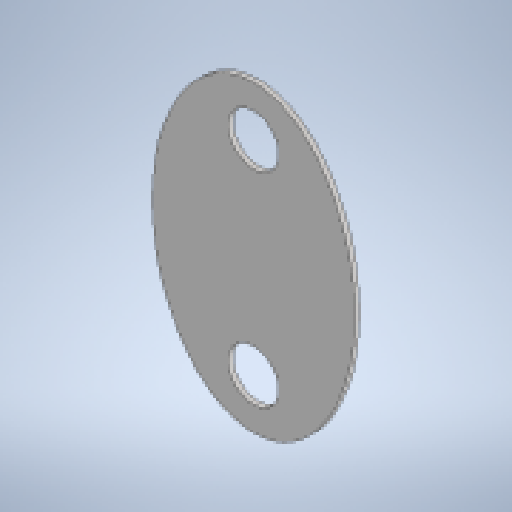
# Autodesk Inventor part: нижний эллипс тела
Saved by Autodesk Inventor 2023.1 (Build 271208000, 208)
## iProperties
Created: 2024-11-21
Part Number: нижний эллипс тела
Material: Типовые
Document SubType Name: Modeling
Designer: DELL
Density: 1 g/cm^3
Appearance: По умолчанию
Author: DELL
Autodesk Inventor part; units mm, degrees
ref_plane "YZ Plane" through (0, 0, 0) normal (1, 0, 0) x (0, 1, 0)
ref_plane "XZ Plane" through (0, 0, 0) normal (0, 1, 0) x (-1, 0, 0)
ref_plane "XY Plane" through (0, 0, 0) normal (0, 0, 1) x (1, 0, 0)
sketch "Эскиз1" plane through (0, 0, 0) normal (0, 0, 1) x (1, 0, 0)
  line L0 (2.6725, 99.2298) -> (22.6725, -99.2298) construction
  ellipse E0 centre (12.6725, 0) end of major axis (12.6725, -120) minor radius 80
  circle A0 centre (0, 225.3213) radius 4 construction
  circle A1 centre (0, -225.3213) radius 4 construction
  arc A2 (-125.6303, -24.4298) -> (-125.6303, -42.4298) centre (-125.6303, -33.4298) ccw construction
  line L1 (-125.6303, -24.4298) -> (-77.5364, -24.4298) construction
  arc A3 (-77.5364, -42.4298) -> (-77.5364, -24.4298) centre (-77.5364, -33.4298) ccw construction
  line L2 (-77.5364, -42.4298) -> (-125.6303, -42.4298) construction
  line L3 (-25, -17) -> (-32, -17) construction
  line L4 (-32, -17) -> (-32, -7) construction
  line L5 (-32, -7) -> (-25, -7) construction
  line L6 (-25, -7) -> (-25, -17) construction
  line L7 (-125.6303, 42.4298) -> (-77.5364, 42.4298) construction
  arc A4 (-77.5364, 24.4298) -> (-77.5364, 42.4298) centre (-77.5364, 33.4298) ccw construction
  line L8 (-77.5364, 24.4298) -> (-125.6303, 24.4298) construction
  arc A5 (-125.6303, 42.4298) -> (-125.6303, 24.4298) centre (-125.6303, 33.4298) ccw construction
  line L9 (-125, 7) -> (-132, 7) construction
  line L10 (-132, 7) -> (-132, 17) construction
  line L11 (-132, 17) -> (-125, 17) construction
  line L12 (-125, 17) -> (-125, 7) construction
  circle A6 centre (159.3262, -159.3262) radius 4 construction
  circle A7 centre (-159.3262, -159.3262) radius 4 construction
  line L13 (22.6725, -100.7298) -> (2.6725, -100.7298) construction
  line L14 (2.6725, -100.7298) -> (2.6725, -60.7298) construction
  line L15 (2.6725, -60.7298) -> (22.6725, -60.7298) construction
  line L16 (22.6725, -60.7298) -> (22.6725, -100.7298) construction
  circle A8 centre (-159.3262, 159.3262) radius 4 construction
  circle A9 centre (225.3213, 0) radius 4 construction
  line L17 (-32, 17) -> (-25, 17) construction
  line L18 (-25, 17) -> (-25, 7) construction
  line L19 (-25, 7) -> (-32, 7) construction
  line L20 (-32, 7) -> (-32, 17) construction
  line L21 (-75, -17) -> (-82, -17) construction
  line L22 (-82, -17) -> (-82, -7) construction
  line L23 (-82, -7) -> (-75, -7) construction
  line L24 (-75, -7) -> (-75, -17) construction
  line L25 (-125, -17) -> (-132, -17) construction
  line L26 (-132, -17) -> (-132, -7) construction
  line L27 (-132, -7) -> (-125, -7) construction
  line L28 (-125, -7) -> (-125, -17) construction
  line L29 (-75, 7) -> (-82, 7) construction
  line L30 (-82, 7) -> (-82, 17) construction
  line L31 (-82, 17) -> (-75, 17) construction
  line L32 (-75, 17) -> (-75, 7) construction
  circle A10 centre (159.3262, 159.3262) radius 4 construction
  circle A11 centre (-225.3213, 0) radius 4 construction
  line L33 (22.6725, 60.7298) -> (2.6725, 60.7298) construction
  line L34 (2.6725, 60.7298) -> (2.6725, 100.7298) construction
  line L35 (2.6725, 100.7298) -> (22.6725, 100.7298) construction
  line L36 (22.6725, 100.7298) -> (22.6725, 60.7298) construction
  circle A12 centre (-104.2556, 141.9298) radius 1.5 construction
  line L37 (-71.1919, 138.9298) -> (-71.1919, 144.9298) construction
  line L38 (-71.1919, 144.9298) -> (-57.9061, 144.9298) construction
  line L39 (-57.9061, 144.9298) -> (-57.9061, 138.9298) construction
  line L40 (-57.9061, 138.9298) -> (-71.1919, 138.9298) construction
  line L41 (-97.7633, 55.9298) -> (-97.7633, 61.9298) construction
  line L42 (-97.7633, 61.9298) -> (-84.4776, 61.9298) construction
  line L43 (-84.4776, 61.9298) -> (-84.4776, 55.9298) construction
  line L44 (-84.4776, 55.9298) -> (-97.7633, 55.9298) construction
  circle A13 centre (-77.5336, 58.9298) radius 1.5 construction
  line L45 (-101.4061, 113.2631) -> (-101.4061, 87.5965) construction
  line L46 (-101.4061, 87.5965) -> (-107.4061, 87.5965) construction
  line L47 (-107.4061, 87.5965) -> (-107.4061, 113.2631) construction
  line L48 (-107.4061, 113.2631) -> (-101.4061, 113.2631) construction
  line L49 (83.8167, 100.7298) -> (83.8167, 106.7298) construction
  line L50 (83.8167, 106.7298) -> (96.6738, 106.7298) construction
  line L51 (96.6738, 106.7298) -> (96.6738, 100.7298) construction
  line L52 (96.6738, 100.7298) -> (83.8167, 100.7298) construction
  line L53 (109.531, 100.7298) -> (109.531, 106.7298) construction
  line L54 (109.531, 106.7298) -> (122.3881, 106.7298) construction
  line L55 (122.3881, 106.7298) -> (122.3881, 100.7298) construction
  line L56 (122.3881, 100.7298) -> (109.531, 100.7298) construction
  circle A14 centre (77.3881, 103.7298) radius 1.5 construction
  circle A15 centre (129.1261, 141.9298) radius 1.5 construction
  line L57 (-84.4776, -138.9298) -> (-84.4776, -144.9298) construction
  line L58 (-84.4776, -144.9298) -> (-97.7633, -144.9298) construction
  line L59 (-97.7633, -144.9298) -> (-97.7633, -138.9298) construction
  line L60 (-97.7633, -138.9298) -> (-84.4776, -138.9298) construction
  line L61 (-71.1919, -55.9298) -> (-57.9061, -55.9298) construction
  line L62 (-57.9061, -55.9298) -> (-57.9061, -61.9298) construction
  line L63 (-57.9061, -61.9298) -> (-71.1919, -61.9298) construction
  line L64 (-71.1919, -61.9298) -> (-71.1919, -55.9298) construction
  circle A16 centre (-77.5336, -141.9298) radius 1.5 construction
  line L65 (135.2452, -100.7298) -> (148.1024, -100.7298) construction
  line L66 (148.1024, -100.7298) -> (148.1024, -106.7298) construction
  line L67 (148.1024, -106.7298) -> (135.2452, -106.7298) construction
  line L68 (135.2452, -106.7298) -> (135.2452, -100.7298) construction
  line L69 (70.9595, -106.7298) -> (58.1024, -106.7298) construction
  line L70 (58.1024, -106.7298) -> (58.1024, -100.7298) construction
  line L71 (58.1024, -100.7298) -> (70.9595, -100.7298) construction
  line L72 (70.9595, -100.7298) -> (70.9595, -106.7298) construction
  circle A17 centre (77.3881, -141.9298) radius 1.5 construction
  line L73 (122.3881, -106.7298) -> (109.531, -106.7298) construction
  line L74 (109.531, -106.7298) -> (109.531, -100.7298) construction
  line L75 (109.531, -100.7298) -> (122.3881, -100.7298) construction
  line L76 (122.3881, -100.7298) -> (122.3881, -106.7298) construction
  line L77 (96.6738, -100.7298) -> (96.6738, -106.7298) construction
  line L78 (96.6738, -106.7298) -> (83.8167, -106.7298) construction
  line L79 (83.8167, -106.7298) -> (83.8167, -100.7298) construction
  line L80 (83.8167, -100.7298) -> (96.6738, -100.7298) construction
  circle A18 centre (103.2571, -141.9298) radius 1.5 construction
  line L81 (135.2452, -144.9298) -> (135.2452, -138.9298) construction
  line L82 (135.2452, -138.9298) -> (148.1024, -138.9298) construction
  line L83 (148.1024, -138.9298) -> (148.1024, -144.9298) construction
  line L84 (148.1024, -144.9298) -> (135.2452, -144.9298) construction
  circle A19 centre (-77.5336, -58.9298) radius 1.5 construction
  circle A20 centre (-104.2556, -141.9298) radius 1.5 construction
  line L85 (-107.4061, -113.2631) -> (-107.4061, -87.5965) construction
  line L86 (-107.4061, -87.5965) -> (-101.4061, -87.5965) construction
  line L87 (-101.4061, -87.5965) -> (-101.4061, -113.2631) construction
  line L88 (-101.4061, -113.2631) -> (-107.4061, -113.2631) construction
  line L89 (-111.049, -138.9298) -> (-111.049, -144.9298) construction
  line L90 (-111.049, -144.9298) -> (-124.3347, -144.9298) construction
  line L91 (-124.3347, -144.9298) -> (-124.3347, -138.9298) construction
  line L92 (-124.3347, -138.9298) -> (-111.049, -138.9298) construction
  circle A21 centre (129.1261, 103.7298) radius 1.5 construction
  circle A22 centre (77.3881, 141.9298) radius 1.5 construction
  line L93 (96.6738, 138.9298) -> (83.8167, 138.9298) construction
  line L94 (83.8167, 138.9298) -> (83.8167, 144.9298) construction
  line L95 (83.8167, 144.9298) -> (96.6738, 144.9298) construction
  line L96 (96.6738, 144.9298) -> (96.6738, 138.9298) construction
  line L97 (135.2452, 100.7298) -> (135.2452, 106.7298) construction
  line L98 (135.2452, 106.7298) -> (148.1024, 106.7298) construction
  line L99 (148.1024, 106.7298) -> (148.1024, 100.7298) construction
  line L100 (148.1024, 100.7298) -> (135.2452, 100.7298) construction
  line L101 (-150.9061, 55.9298) -> (-150.9061, 61.9298) construction
  line L102 (-150.9061, 61.9298) -> (-137.6204, 61.9298) construction
  line L103 (-137.6204, 61.9298) -> (-137.6204, 55.9298) construction
  line L104 (-137.6204, 55.9298) -> (-150.9061, 55.9298) construction
  circle A23 centre (-104.2556, 58.9298) radius 1.5 construction
  circle A24 centre (-130.9776, 141.9298) radius 1.5 construction
  circle A25 centre (-77.5336, 141.9298) radius 1.5 construction
  line L105 (-124.3347, 55.9298) -> (-124.3347, 61.9298) construction
  line L106 (-124.3347, 61.9298) -> (-111.049, 61.9298) construction
  line L107 (-111.049, 61.9298) -> (-111.049, 55.9298) construction
  line L108 (-111.049, 55.9298) -> (-124.3347, 55.9298) construction
  line L109 (-124.3347, 138.9298) -> (-124.3347, 144.9298) construction
  line L110 (-124.3347, 144.9298) -> (-111.049, 144.9298) construction
  line L111 (-111.049, 144.9298) -> (-111.049, 138.9298) construction
  line L112 (-111.049, 138.9298) -> (-124.3347, 138.9298) construction
  line L113 (-97.7633, 144.9298) -> (-84.4776, 144.9298) construction
  line L114 (-84.4776, 144.9298) -> (-84.4776, 138.9298) construction
  line L115 (-84.4776, 138.9298) -> (-97.7633, 138.9298) construction
  line L116 (-97.7633, 138.9298) -> (-97.7633, 144.9298) construction
  line L117 (135.2452, 144.9298) -> (148.1024, 144.9298) construction
  line L118 (148.1024, 144.9298) -> (148.1024, 138.9298) construction
  line L119 (148.1024, 138.9298) -> (135.2452, 138.9298) construction
  line L120 (135.2452, 138.9298) -> (135.2452, 144.9298) construction
  line L121 (70.9595, 144.9298) -> (70.9595, 138.9298) construction
  line L122 (70.9595, 138.9298) -> (58.1024, 138.9298) construction
  line L123 (58.1024, 138.9298) -> (58.1024, 144.9298) construction
  line L124 (58.1024, 144.9298) -> (70.9595, 144.9298) construction
  circle A26 centre (103.2571, 103.7298) radius 1.5 construction
  line L125 (-137.6204, -144.9298) -> (-150.9061, -144.9298) construction
  line L126 (-150.9061, -144.9298) -> (-150.9061, -138.9298) construction
  line L127 (-150.9061, -138.9298) -> (-137.6204, -138.9298) construction
  line L128 (-137.6204, -138.9298) -> (-137.6204, -144.9298) construction
  line L129 (-71.1919, -138.9298) -> (-57.9061, -138.9298) construction
  line L130 (-57.9061, -138.9298) -> (-57.9061, -144.9298) construction
  line L131 (-57.9061, -144.9298) -> (-71.1919, -144.9298) construction
  line L132 (-71.1919, -144.9298) -> (-71.1919, -138.9298) construction
  line L133 (-84.4776, -55.9298) -> (-84.4776, -61.9298) construction
  line L134 (-84.4776, -61.9298) -> (-97.7633, -61.9298) construction
  line L135 (-97.7633, -61.9298) -> (-97.7633, -55.9298) construction
  line L136 (-97.7633, -55.9298) -> (-84.4776, -55.9298) construction
  circle A27 centre (-104.2556, -58.9298) radius 1.5 construction
  line L137 (58.1024, -144.9298) -> (58.1024, -138.9298) construction
  line L138 (58.1024, -138.9298) -> (70.9595, -138.9298) construction
  line L139 (70.9595, -138.9298) -> (70.9595, -144.9298) construction
  line L140 (70.9595, -144.9298) -> (58.1024, -144.9298) construction
  circle A28 centre (129.1261, -141.9298) radius 1.5 construction
  circle A29 centre (103.2571, -103.7298) radius 1.5 construction
  line L141 (109.531, -144.9298) -> (109.531, -138.9298) construction
  line L142 (109.531, -138.9298) -> (122.3881, -138.9298) construction
  line L143 (122.3881, -138.9298) -> (122.3881, -144.9298) construction
  line L144 (122.3881, -144.9298) -> (109.531, -144.9298) construction
  circle A30 centre (77.3881, -103.7298) radius 1.5 construction
  circle A31 centre (129.1261, -103.7298) radius 1.5 construction
  line L145 (83.8167, -144.9298) -> (83.8167, -138.9298) construction
  line L146 (83.8167, -138.9298) -> (96.6738, -138.9298) construction
  line L147 (96.6738, -138.9298) -> (96.6738, -144.9298) construction
  line L148 (96.6738, -144.9298) -> (83.8167, -144.9298) construction
  circle A32 centre (-130.9776, -141.9298) radius 1.5 construction
  line L149 (-124.3347, -55.9298) -> (-111.049, -55.9298) construction
  line L150 (-111.049, -55.9298) -> (-111.049, -61.9298) construction
  line L151 (-111.049, -61.9298) -> (-124.3347, -61.9298) construction
  line L152 (-124.3347, -61.9298) -> (-124.3347, -55.9298) construction
  circle A33 centre (-130.9776, -58.9298) radius 1.5 construction
  line L153 (-150.9061, -55.9298) -> (-137.6204, -55.9298) construction
  line L154 (-137.6204, -55.9298) -> (-137.6204, -61.9298) construction
  line L155 (-137.6204, -61.9298) -> (-150.9061, -61.9298) construction
  line L156 (-150.9061, -61.9298) -> (-150.9061, -55.9298) construction
  circle A34 centre (103.2571, 141.9298) radius 1.5 construction
  line L157 (58.1024, 106.7298) -> (70.9595, 106.7298) construction
  line L158 (70.9595, 106.7298) -> (70.9595, 100.7298) construction
  line L159 (70.9595, 100.7298) -> (58.1024, 100.7298) construction
  line L160 (58.1024, 100.7298) -> (58.1024, 106.7298) construction
  line L161 (109.531, 144.9298) -> (122.3881, 144.9298) construction
  line L162 (122.3881, 144.9298) -> (122.3881, 138.9298) construction
  line L163 (122.3881, 138.9298) -> (109.531, 138.9298) construction
  line L164 (109.531, 138.9298) -> (109.531, 144.9298) construction
  line L165 (-71.1919, 61.9298) -> (-57.9061, 61.9298) construction
  line L166 (-57.9061, 61.9298) -> (-57.9061, 55.9298) construction
  line L167 (-57.9061, 55.9298) -> (-71.1919, 55.9298) construction
  line L168 (-71.1919, 55.9298) -> (-71.1919, 61.9298) construction
  line L169 (-137.6204, 138.9298) -> (-150.9061, 138.9298) construction
  line L170 (-150.9061, 138.9298) -> (-150.9061, 144.9298) construction
  line L171 (-150.9061, 144.9298) -> (-137.6204, 144.9298) construction
  line L172 (-137.6204, 144.9298) -> (-137.6204, 138.9298) construction
  circle A35 centre (-130.9776, 58.9298) radius 1.5 construction
  circle A36 centre (0, 0) radius 240 construction
  line L173 (2.6725, -100.7298) -> (22.6725, -60.7298) construction
  line L174 (22.6725, 100.7298) -> (2.6725, 60.7298) construction
  circle A37 centre (12.6725, -80.7298) radius 20
  circle A38 centre (12.6725, 80.7298) radius 20
  dimension "d2" = 120
  dimension "d3" = 80
  constraints: 6 end point, 3 midpoint, 2 centre point, 1 parallel, 4 other
extrude "Выдавливание1" add sketch "Эскиз1" against normal blind 4
